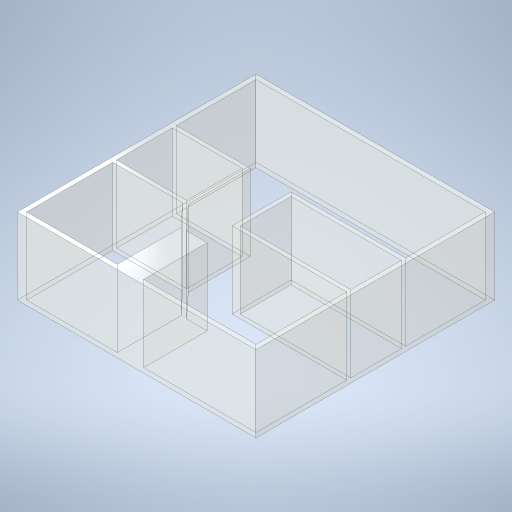
# Autodesk Inventor part: Existing_Kitchen_And_Dining_Room
Saved by Autodesk Inventor 2024 (Build 280153000, 153)
## iProperties
Created: 2023-04-15
Part Number: Existing_Kitchen_And_Dining_Room
Material: Glass
Document SubType Name: Modeling
Designer: Tom
Density: 2.18 g/cm^3
Appearance: Clear
Author: Tom
Autodesk Inventor part; units mm, degrees
ref_plane "YZ Plane" through (0, 0, 0) normal (1, 0, 0) x (0, 1, 0)
ref_plane "XZ Plane" through (0, 0, 0) normal (0, 1, 0) x (-1, 0, 0)
ref_plane "XY Plane" through (0, 0, 0) normal (0, 0, 1) x (1, 0, 0)
sketch "Sketch1" plane through (0, 0, 0) normal (0, 1, 0) x (-1, 0, 0)
  line L0 (149.225, -7470.775) -> (149.225, 149.225)
  line L1 (149.225, 149.225) -> (-7470.775, 149.225)
  line L2 (-7470.775, 149.225) -> (-7470.775, -7470.775)
  line L3 (-7470.775, -7470.775) -> (149.225, -7470.775)
  line L4 (149.225, -2876.55) -> (149.225, -3028.95)
  line L5 (0, 0) -> (0, -7321.55)
  line L6 (0, -7321.55) -> (-7321.55, -7321.55)
  line L7 (-7321.55, -7321.55) -> (-7321.55, 0)
  line L8 (-7321.55, 0) -> (0, 0)
  line L9 (0, -2743.2) -> (-2235.2, -2743.2)
  line L10 (-2235.2, -2743.2) -> (-2895.6, -2032)
  line L11 (-2895.6, -2032) -> (-2895.6, 0)
  line L12 (0, -2873.375) -> (-2235.2, -2873.375)
  line L13 (-2235.2, -2873.375) -> (-2235.2, -4645.3435)
  line L14 (-2235.2, -4645.3435) -> (0, -4645.3435)
  line L15 (0, -4775.5185) -> (-2365.375, -4775.5185)
  line L16 (-2365.375, -4775.5185) -> (-2365.375, -2794.3185)
  line L17 (-2365.375, -2794.3185) -> (-3073.2421, -2032)
  line L18 (-3073.2421, -2032) -> (-3733.6421, -2032)
  line L19 (-3733.6421, -2032) -> (-3733.6421, 0)
  line L20 (-7321.55, -3025.775) -> (-3794.125, -3025.775)
  line L21 (-3794.125, -3025.775) -> (-3794.125, -4645.3435)
  line L22 (-3663.95, -4775.5185) -> (-3663.95, -2895.6)
  line L23 (-3663.95, -2895.6) -> (-7321.55, -2895.6)
  line L24 (-3663.95, -4775.5185) -> (-7321.55, -4775.5185)
  line L25 (-7321.55, -4645.3435) -> (-3794.125, -4645.3435)
  dimension "d34" = 7620
  dimension "d37" = 149.225
  dimension "d38" = 7620
  dimension "d39" = 2743.2
  dimension "d40" = 2032
  dimension "d42" = 2235.2
  dimension "d44" = 130.175
  dimension "d47" = 130.175
  dimension "d48" = 1981.2
  dimension "d49" = 130.175
  dimension "d50" = 130.175
  dimension "d52" = 2032
  dimension "d53" = 2895.6
  dimension "d55" = 130.175
  dimension "d57" = 2895.6
  dimension "d58" = 130.175
  dimension "d59" = 3657.6
  dimension "d62" = 660.4
  constraints: 52 end point, 12 perpendicular, 10 point on line, 6 horizontal, 3 collinear, 3 parallel, 1 coincident, 3 other
  measures "d34" distance of L1.end L2.end
  measures "d37" distance between parallel lines of L0 L5
  measures "d38" distance of L2.end L0.start
  measures "d39" distance between parallel lines of L8 L9
  measures "d40" distance of L10.end L11.end
  measures "d42" distance of L12.start L12.end
  measures "d44" distance between parallel lines of L9 L12
  measures "d47" distance between parallel lines of L13 L16
  measures "d48" distance of L15.end L16.end
  measures "d49" distance between parallel lines of L15 L14
  measures "d50" distance between parallel lines of L10 L17
  measures "d52" distance of L18.end L19.end
  measures "d53" distance between parallel lines of L5 L11
  measures "d55" distance between parallel lines of L21 L22
  measures "d57" distance between parallel lines of L8 L23
  measures "d58" distance between parallel lines of L20 L23
  measures "d59" distance of L22.end L23.end
  measures "d62" distance of L17.end L18.end
extrude "Extrusion1" add sketch "Sketch1" along normal blind 2438.4 contours L3 L2 L1 L0 | L5 L12 L13 L14 L15 L16 L17 L18 L19 L8 L11 L10 L9 | L23 L22 L24 L7 L25 L21 L20
body "Solid1"
